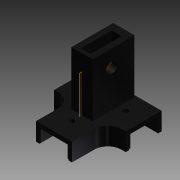
# Autodesk Inventor part: T-top Bearing Hoder
Saved by Autodesk Inventor 2015 (Build 190159000, 159)
## iProperties
Created: 2013-08-27
Part Number: T-top Bearing Hoder
Material: PC/ABS Plastic
Document SubType Name: Modeling
Designer: jesse
Mass: 3.57334 g
Surface Area: 72.7881 cm^2
Volume: 10.0017 cm^3
Density: 0.357273 g/cm^3
Appearance: Glossy - Black
Author: Jesse Stevenson
Autodesk Inventor part; units mm, degrees
ref_plane "YZ Plane" through (0, 0, 0) normal (1, 0, 0) x (0, 1, 0)
ref_plane "XZ Plane" through (0, 0, 0) normal (0, 1, 0) x (-1, 0, 0)
ref_plane "XY Plane" through (0, 0, 0) normal (0, 0, 1) x (1, 0, 0)
sketch "Sketch1" plane through (0, 0, 0) normal (0, 0, 1) x (1, 0, 0)
  line L0 (-12.7, -12.7) -> (12.7, -12.7)
  line L1 (12.7, -12.7) -> (12.7, 12.7)
  line L2 (12.7, 12.7) -> (-12.7, 12.7)
  line L3 (-12.7, 12.7) -> (-12.7, -12.7)
  line L4 (-12.7, -12.7) -> (12.7, 12.7) construction
  line L5 (12.7, -12.7) -> (-12.7, 12.7) construction
  point P0 (0, 0)
  dimension "d0" = 25.4
  dimension "d1" = 25.4
  constraints: 12 end point, 2 midpoint, 2 parallel, 1 horizontal, 1 perpendicular
  measures "d0" distance of L2.end L1.end
  measures "d1" distance of L1.end L0.end
extrude "Extrusion1" add sketch "Sketch1" along normal blind 50.8
sketch "Sketch2" plane through (12.7, -12.7, 0) normal (1, 0, 0) x (0, 0, -1)
  line L0 (0, 0) -> (-50.8, 0) projected
  line L1 (0, 25.4) -> (-25.4, 25.4)
  line L2 (-25.4, 25.4) -> (-25.4, 0)
  line L3 (-25.4, 0) -> (0, 0)
  line L4 (0, 0) -> (0, 25.4)
  point P0 (0, 12.7)
  constraints: 8 end point, 2 parallel, 1 horizontal, 1 midpoint, 1 perpendicular
extrude "Extrusion2" add sketch "Sketch2" along normal blind 12.7
sketch "Sketch4" plane through (-12.7, -12.7, 0) normal (-1, 0, 0) x (0, 0, 1)
  line L0 (0, 25.4) -> (0, 0) projected
  line L1 (0, 0) -> (50.8, 0) projected
  line L2 (0, 25.4) -> (25.4, 25.4)
  line L3 (25.4, 25.4) -> (25.4, 0)
  line L4 (25.4, 0) -> (0, 0)
  line L5 (0, 0) -> (0, 25.4)
  point P0 (0, 12.7)
  constraints: 8 end point, 2 parallel, 1 horizontal, 1 midpoint, 1 perpendicular
extrude "Extrusion3" add sketch "Sketch4" along normal blind 12.7
sketch "Sketch5" plane through (0, 0, 50.8) normal (0, 0, 1) x (1, 0, 0)
  line L0 (-9.525, 9.525) -> (9.525, 9.525)
  line L1 (9.525, 9.525) -> (9.525, -9.525)
  line L2 (9.525, -9.525) -> (-9.525, -9.525)
  line L3 (-9.525, -9.525) -> (-9.525, 9.525)
  line L4 (-9.525, 9.525) -> (9.525, -9.525) construction
  line L5 (9.525, 9.525) -> (-9.525, -9.525) construction
  point P0 (0, 0)
  dimension "d8" = 19.05
  dimension "d9" = 19.05
  constraints: 12 end point, 2 midpoint, 2 parallel, 1 horizontal, 1 perpendicular
  measures "d8" distance of L1.end L2.end
  measures "d9" distance of L0.end L1.end
extrude "Extrusion4" cut sketch "Sketch5" against normal blind 44.45
sketch "Sketch6" plane through (25.4, -12.7, 0) normal (1, 0, 0) x (0, 0, -1)
  line L0 (-22.225, 22.225) -> (-3.175, 22.225)
  line L1 (-3.175, 22.225) -> (-3.175, 3.175)
  line L2 (-3.175, 3.175) -> (-22.225, 3.175)
  line L3 (-22.225, 3.175) -> (-22.225, 22.225)
  line L4 (-22.225, 22.225) -> (-3.175, 3.175) construction
  line L5 (-3.175, 22.225) -> (-22.225, 3.175) construction
  point P0 (0, 12.7)
  point P1 (-12.7, 12.7)
  dimension "d12" = 19.05
  dimension "d13" = 19.05
  constraints: 12 end point, 2 midpoint, 2 parallel, 1 horizontal, 1 perpendicular
  measures "d12" distance of L1.end L2.end
  measures "d13" distance of L0.end L1.end
extrude "Extrusion5" cut sketch "Sketch6" against normal through all
split "Split1" plane through (0, 0, 0) removes the side toward (0, -1, 0)
lip "Lip1" kind groove height 0.762 width 0.762 edges at (9.525, 0, 36.5125) (17.4625, 0, 22.225) guide face at (10.5833, 0, 32.8083)
lip "Lip2" kind groove height 0.762 width 0.762 edges at (-9.525, 0, 36.5125) (-17.4625, 0, 22.225) guide face at (-10.5833, 0, 32.8083)
lip "Lip3" kind groove height 0.762 width 0.762 edges at (0, 0, 3.175) guide face at (-8.4667, 0, 1.0583)
sketch "Sketch7" plane through (-12.7, 12.7, 50.8) normal (0, 1, 0) x (1, 0, 0)
  line L0 (-12.7, 50.8) -> (38.1, 50.8) projected
  line L1 (-12.7, 25.4) -> (-12.7, 50.8) projected
  line L2 (25.4, 0) -> (0, 0) projected
  line L3 (38.1, 50.8) -> (38.1, 25.4) projected
  line L4 (12.7, 50.8) -> (12.7, 0) construction
  line L5 (-12.7, 38.1) -> (38.1, 38.1) construction
  line L6 (25.4, 25.4) -> (25.4, 50.8) construction
  circle A0 centre (0, 38.1) radius 1.7907
  circle A1 centre (25.4, 38.1) radius 1.7907
  circle A2 centre (12.7, 12.7) radius 1.7907
  dimension "d34" = 3.5814
  constraints: 6 end point, 4 midpoint, 3 centre point, 3 point on line, 2 equal radius, 1 perpendicular
  measures "d34" diameter of A0
extrude "Extrusion6" cut sketch "Sketch7" against normal through all
fillet "Fillet1" radius 9.525 2 edges at (-12.7, 6.35, 25.4) (12.7, 6.35, 25.4)
sketch "Sketch8" plane through (-12.7, 12.7, 50.8) normal (0, 1, 0) x (1, 0, 0)
  circle A0 centre (25.4, 38.1) radius 1.7907 construction
  circle A1 centre (0, 38.1) radius 1.7907 construction
  circle A2 centre (12.7, 12.7) radius 1.7907 projected
  line L0 (-12.7, 50.8) -> (38.1, 50.8) projected
  line L1 (-12.7, 25.4) -> (-12.7, 50.8) projected
  line L2 (-9.525, 25.4) -> (-12.7, 25.4) projected
  arc A3 (0, 15.875) -> (-9.525, 25.4) centre (-9.525, 15.875) ccw projected
  line L3 (0, 15.875) -> (0, 0) projected
  line L4 (25.4, 0) -> (0, 0) projected
  line L5 (25.4, 15.875) -> (25.4, 0) projected
  arc A4 (34.925, 25.4) -> (25.4, 15.875) centre (34.925, 15.875) ccw projected
  line L6 (34.925, 25.4) -> (38.1, 25.4) projected
  line L7 (38.1, 50.8) -> (38.1, 25.4) projected
  line L8 (38.1, 50.8) -> (38.1, 25.4) construction
  line L9 (38.1, 38.1) -> (-12.7, 38.1) construction
  line L10 (-12.7, 47.625) -> (-12.7, 28.575) construction
  line L11 (12.7, 38.1) -> (12.7, 49.4529) construction
  line L12 (12.7, 32.4235) -> (20.2287, 32.4235) construction
  line L13 (12.7, 32.4235) -> (5.1713, 32.4235) construction
  line L14 (12.7, 43.7765) -> (20.2287, 43.7765) construction
  line L15 (12.7, 43.7765) -> (5.1713, 43.7765) construction
  line L16 (20.2287, 49.4529) -> (5.1713, 49.4529)
  line L17 (5.1713, 49.4529) -> (5.1713, 19.752)
  line L18 (5.1713, 19.752) -> (20.2287, 19.752)
  line L19 (20.2287, 19.752) -> (20.2287, 49.4529)
  point P0 (12.7, 50.8)
  constraints: 20 end point, 5 horizontal, 5 midpoint, 3 equal length, 2 parallel, 2 point on line, 1 perpendicular, 1 vertical
extrude "Extrusion7" add sketch "Sketch8" along normal blind 25.4 contours L19 L18 L17 L16
ref_plane "Work Plane1" through (0, 12.7, 31.048) normal (1, 0, 0) x (0, 0, -1)
sketch "Sketch9" plane through (0, 12.7, 31.048) normal (1, 0, 0) x (0, 0, -1)
  circle A0 centre (13.6363, 26.2767) radius 10.95 projected
  point P0 (31.048, -12.7)
ref_plane "Work Plane2" through (3.5298, 23.701, 2.136) normal (1, 0, 0) x (0, 0.8135499, -0.5814951)
extrude "Extrusion8" cut sketch "Sketch9" along normal up to surface (3.5298 mm away)
sketch "Sketch10" plane through (0, 12.7, 31.048) normal (1, 0, 0) x (0, 0, -1)
  circle A0 centre (13.6363, 26.2767) radius 4 construction
  circle A1 centre (13.6363, 26.2767) radius 10.95 projected
  point P0 (31.048, -12.7)
ref_plane "Work Plane3" through (-3.3702, 23.701, 2.136) normal (-1, 0, 0) x (0, 0.5814951, 0.8135499)
extrude "Extrusion9" cut sketch "Sketch10" against normal up to surface (3.3702 mm away)
sketch "Sketch11" plane through (-12.7, 38.1, 50.8) normal (0, 1, 0) x (1, 0, 0)
  line L0 (20.2287, 49.4529) -> (5.1713, 49.4529) projected
  line L1 (5.1713, 49.4529) -> (5.1713, 19.752) projected
  line L2 (5.1713, 19.752) -> (20.2287, 19.752) projected
  line L3 (20.2287, 19.752) -> (20.2287, 49.4529) projected
  line L4 (16.2298, 22.4735) -> (9.3298, 22.4735) projected
  line L5 (9.3298, 22.4735) -> (9.3298, 44.3031) projected
  line L6 (9.3298, 44.3031) -> (16.2298, 44.3031) projected
  line L7 (16.2298, 44.3031) -> (16.2298, 22.4735) projected
  point P0 (12.7, 50.8)
extrude "Extrusion10" add sketch "Sketch11" along normal blind 12.7
sketch "Sketch12" plane through (7.5287, 12.7, 31.048) normal (1, 0, 0) x (0, 0, -1)
  circle A0 centre (13.6363, 26.2767) radius 6.7
  point P0 (31.048, -12.7)
  dimension "d47" = 13.4
  constraints: 1 centre point
  measures "d47" diameter of A0
extrude "Extrusion11" cut sketch "Sketch12" against normal through all
sketch "Sketch13" plane through (7.5287, 12.7, 1.3471) normal (0, 0, -1) x (-1, 0, 0)
  line L0 (15.0573, 0) -> (0, 0) projected
  line L1 (15.0573, 0) -> (15.0573, 38.1) projected
  line L2 (0, 38.1) -> (15.0573, 38.1) projected
  line L3 (0, 0) -> (0, 38.1) projected
  point P0 (7.5287, -12.7)
extrude "Extrusion12" add sketch "Sketch13" along normal up to surface (1.3471 mm away)
body "Solid1"
